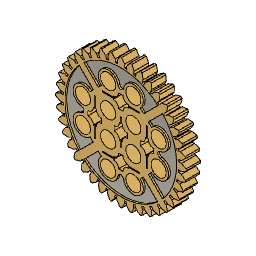
Gear_v1 (Autodesk Fusion 360 design; units mm, degrees)
Autodesk Fusion 360 part; units mm, degrees
(part 1 of 2)
sketch "Sketch1" plane through (0, 0, 0) normal (0, 1, 0) x (1, 0, 0) in component "Component"
sketch "Sketch1 (2)" plane through (0, 0, 0) normal (0, 1, 0) x (1, 0, 0)
  circle A0 centre (36.5707, -36.5204) radius 32.2395
  line L0 (34.5837, -4.281) -> (34.5837, -2.63)
  line L1 (34.5837, -2.63) -> (36.0971, -0.1323)
  line L2 (36.0971, -0.1323) -> (37.0337, -0.1323)
  line L3 (37.0337, -0.1323) -> (38.5022, -2.6935)
  line L4 (38.5022, -2.6935) -> (38.5022, -4.3286)
  line L5 (38.5022, -68.8049) -> (38.5022, -70.4559)
  line L6 (38.5022, -70.4559) -> (36.9888, -72.9536)
  line L7 (36.9888, -72.9536) -> (36.0521, -72.9536)
  line L8 (36.0521, -72.9536) -> (34.5837, -70.3924)
  line L9 (34.5837, -70.3924) -> (34.5837, -68.7599)
  line L10 (29.5619, -4.9848) -> (29.3026, -3.3549)
  line L11 (29.3026, -3.3549) -> (30.4059, -0.6509)
  line L12 (30.4059, -0.6509) -> (31.332, -0.5027)
  line L13 (31.332, -0.5027) -> (33.184, -2.8046)
  line L14 (33.184, -2.8046) -> (33.438, -4.4185)
  line L15 (43.5266, -68.1011) -> (43.7833, -69.7309)
  line L16 (43.7833, -69.7309) -> (42.6799, -72.4376)
  line L17 (42.6799, -72.4376) -> (41.7539, -72.5831)
  line L18 (41.7539, -72.5831) -> (39.9045, -70.2839)
  line L19 (39.9045, -70.2839) -> (39.6478, -68.67)
  line L20 (24.7094, -6.4638) -> (24.2014, -4.8948)
  line L21 (24.2014, -4.8948) -> (24.8682, -2.0532)
  line L22 (24.8682, -2.0532) -> (25.7598, -1.7621)
  line L23 (25.7598, -1.7621) -> (27.9479, -3.7439)
  line L24 (27.9479, -3.7439) -> (28.4506, -5.2996)
  line L25 (48.3764, -66.6221) -> (48.8871, -68.1911)
  line L26 (48.8871, -68.1911) -> (48.2177, -71.0353)
  line L27 (48.2177, -71.0353) -> (47.3287, -71.3237)
  line L28 (47.3287, -71.3237) -> (45.1406, -69.342)
  line L29 (45.1406, -69.342) -> (44.6352, -67.7889)
  line L30 (20.1507, -8.6863) -> (19.4019, -7.2152)
  line L31 (19.4019, -7.2152) -> (19.6162, -4.3021)
  line L32 (19.6162, -4.3021) -> (20.4523, -3.8788)
  line L33 (20.4523, -3.8788) -> (22.9209, -5.4928)
  line L34 (22.9209, -5.4928) -> (23.6643, -6.948)
  line L35 (52.9352, -64.3996) -> (53.684, -65.8707)
  line L36 (53.684, -65.8707) -> (53.4696, -68.7837)
  line L37 (53.4696, -68.7837) -> (52.6362, -69.2097)
  line L38 (52.6362, -69.2097) -> (50.165, -67.5931)
  line L39 (50.165, -67.5931) -> (49.4242, -66.1379)
  line L40 (15.9941, -11.594) -> (15.0257, -10.2579)
  line L41 (15.0257, -10.2579) -> (14.7823, -7.3475)
  line L42 (14.7823, -7.3475) -> (15.539, -6.7971)
  line L43 (15.539, -6.7971) -> (18.2324, -8.0063)
  line L44 (18.2324, -8.0063) -> (19.1929, -9.3292)
  line L45 (57.0918, -61.4918) -> (58.0628, -62.828)
  line L46 (58.0628, -62.828) -> (58.3062, -65.7384)
  line L47 (58.3062, -65.7384) -> (57.5469, -66.2887)
  line L48 (57.5469, -66.2887) -> (54.8561, -65.0796)
  line L49 (54.8561, -65.0796) -> (53.8956, -63.7593)
  line L50 (12.3455, -15.1156) -> (11.1786, -13.9488)
  line L51 (11.1786, -13.9488) -> (10.4828, -11.1125)
  line L52 (10.4828, -11.1125) -> (11.1442, -10.4484)
  line L53 (11.1442, -10.4484) -> (13.9938, -11.221)
  line L54 (13.9938, -11.221) -> (15.1474, -12.3772)
  line L55 (60.743, -57.9702) -> (61.9099, -59.137)
  line L56 (61.9099, -59.137) -> (62.6057, -61.976)
  line L57 (62.6057, -61.976) -> (61.9416, -62.6375)
  line L58 (61.9416, -62.6375) -> (59.0947, -61.8649)
  line L59 (59.0947, -61.8649) -> (57.9385, -60.7086)
  line L60 (9.2922, -19.1638) -> (7.956, -18.1954)
  line L61 (7.956, -18.1954) -> (6.8236, -15.5019)
  line L62 (6.8236, -15.5019) -> (7.3739, -14.7452)
  line L63 (7.3739, -14.7452) -> (10.3108, -15.0627)
  line L64 (10.3108, -15.0627) -> (11.6311, -16.0232)
  line L65 (63.7963, -53.9221) -> (65.1298, -54.8905)
  line L66 (65.1298, -54.8905) -> (66.2623, -57.5839)
  line L67 (66.2623, -57.5839) -> (65.7119, -58.3433)
  line L68 (65.7119, -58.3433) -> (62.7777, -58.0258)
  line L69 (62.7777, -58.0258) -> (61.4548, -57.0653)
  line L70 (6.9083, -23.6432) -> (5.4372, -22.8944)
  line L71 (5.4372, -22.8944) -> (3.8973, -20.41)
  line L72 (3.8973, -20.41) -> (4.3233, -19.5739)
  line L73 (4.3233, -19.5739) -> (7.2734, -19.431)
  line L74 (7.2734, -19.431) -> (8.7286, -20.1718)
  line L75 (66.1802, -49.4453) -> (67.6487, -50.1941)
  line L76 (67.6487, -50.1941) -> (69.1885, -52.6759)
  line L77 (69.1885, -52.6759) -> (68.7626, -53.512)
  line L78 (68.7626, -53.512) -> (65.8151, -53.6575)
  line L79 (65.8151, -53.6575) -> (64.3599, -52.914)
  line L80 (5.2546, -28.4374) -> (3.6856, -27.9268)
  line L81 (3.6856, -27.9268) -> (1.7754, -25.7149)
  line L82 (1.7754, -25.7149) -> (2.0664, -24.8259)
  line L83 (2.0664, -24.8259) -> (4.9556, -24.22)
  line L84 (4.9556, -24.22) -> (6.5088, -24.7253)
  line L85 (67.8339, -44.6484) -> (69.4029, -45.1591)
  line L86 (69.4029, -45.1591) -> (71.3105, -47.371)
  line L87 (71.3105, -47.371) -> (71.0195, -48.2626)
  line L88 (71.0195, -48.2626) -> (68.1302, -48.8659)
  line L89 (68.1302, -48.8659) -> (66.5771, -48.3632)
  line L90 (4.3709, -33.4328) -> (2.7411, -33.1735)
  line L91 (2.7411, -33.1735) -> (0.5106, -31.287)
  line L92 (0.5106, -31.287) -> (0.6562, -30.3609)
  line L93 (0.6562, -30.3609) -> (3.4158, -29.3132)
  line L94 (3.4158, -29.3132) -> (5.0297, -29.5672)
  line L95 (68.7149, -39.6558) -> (70.3448, -39.9124)
  line L96 (70.3448, -39.9124) -> (72.5752, -41.7989)
  line L97 (72.5752, -41.7989) -> (72.4297, -42.7249)
  line L98 (72.4297, -42.7249) -> (69.6701, -43.7727)
  line L99 (69.6701, -43.7727) -> (68.0561, -43.5187)
  line L100 (4.281, -38.5022) -> (2.63, -38.5022)
  line L101 (2.63, -38.5022) -> (0.1323, -36.9888)
  line L102 (0.1323, -36.9888) -> (0.1323, -36.0521)
  line L103 (0.1323, -36.0521) -> (2.6935, -34.5837)
  line L104 (2.6935, -34.5837) -> (4.3286, -34.5837)
  line L105 (68.8049, -34.5837) -> (70.4559, -34.5837)
  line L106 (70.4559, -34.5837) -> (72.9536, -36.0971)
  line L107 (72.9536, -36.0971) -> (72.9536, -37.0337)
  line L108 (72.9536, -37.0337) -> (70.3924, -38.5022)
  line L109 (70.3924, -38.5022) -> (68.7599, -38.5022)
  line L110 (4.9848, -43.5266) -> (3.3549, -43.7833)
  line L111 (3.3549, -43.7833) -> (0.6509, -42.6799)
  line L112 (0.6509, -42.6799) -> (0.5027, -41.7539)
  line L113 (0.5027, -41.7539) -> (2.8046, -39.9045)
  line L114 (2.8046, -39.9045) -> (4.4185, -39.6478)
  line L115 (68.1011, -29.5619) -> (69.7309, -29.3026)
  line L116 (69.7309, -29.3026) -> (72.4376, -30.4059)
  line L117 (72.4376, -30.4059) -> (72.5831, -31.332)
  line L118 (72.5831, -31.332) -> (70.2839, -33.184)
  line L119 (70.2839, -33.184) -> (68.67, -33.438)
  line L120 (6.4638, -48.3764) -> (4.8948, -48.8871)
  line L121 (4.8948, -48.8871) -> (2.0532, -48.2177)
  line L122 (2.0532, -48.2177) -> (1.7621, -47.3287)
  line L123 (1.7621, -47.3287) -> (3.7439, -45.1406)
  line L124 (3.7439, -45.1406) -> (5.2996, -44.6352)
  line L125 (66.6221, -24.7094) -> (68.1911, -24.2014)
  line L126 (68.1911, -24.2014) -> (71.0353, -24.8682)
  line L127 (71.0353, -24.8682) -> (71.3237, -25.7598)
  line L128 (71.3237, -25.7598) -> (69.342, -27.9479)
  line L129 (69.342, -27.9479) -> (67.7889, -28.4506)
  line L130 (8.6863, -52.9352) -> (7.2152, -53.684)
  line L131 (7.2152, -53.684) -> (4.3021, -53.4696)
  line L132 (4.3021, -53.4696) -> (3.8788, -52.6362)
  line L133 (3.8788, -52.6362) -> (5.4928, -50.165)
  line L134 (5.4928, -50.165) -> (6.948, -49.4242)
  line L135 (64.3996, -20.1507) -> (65.8707, -19.4019)
  line L136 (65.8707, -19.4019) -> (68.7837, -19.6162)
  line L137 (68.7837, -19.6162) -> (69.2097, -20.4523)
  line L138 (69.2097, -20.4523) -> (67.5931, -22.9209)
  line L139 (67.5931, -22.9209) -> (66.1379, -23.6643)
  line L140 (11.594, -57.0918) -> (10.2579, -58.0628)
  line L141 (10.2579, -58.0628) -> (7.3475, -58.3062)
  line L142 (7.3475, -58.3062) -> (6.7971, -57.5469)
  line L143 (6.7971, -57.5469) -> (8.0063, -54.8561)
  line L144 (8.0063, -54.8561) -> (9.3292, -53.8956)
  line L145 (61.4918, -15.9941) -> (62.828, -15.0257)
  line L146 (62.828, -15.0257) -> (65.7384, -14.7823)
  line L147 (65.7384, -14.7823) -> (66.2887, -15.539)
  line L148 (66.2887, -15.539) -> (65.0796, -18.2324)
  line L149 (65.0796, -18.2324) -> (63.7593, -19.1929)
  line L150 (15.1156, -60.743) -> (13.9488, -61.9099)
  line L151 (13.9488, -61.9099) -> (11.1125, -62.6057)
  line L152 (11.1125, -62.6057) -> (10.4484, -61.9416)
  line L153 (10.4484, -61.9416) -> (11.221, -59.0947)
  line L154 (11.221, -59.0947) -> (12.3772, -57.9385)
  line L155 (57.9702, -12.3455) -> (59.137, -11.1786)
  line L156 (59.137, -11.1786) -> (61.976, -10.4828)
  line L157 (61.976, -10.4828) -> (62.6375, -11.1442)
  line L158 (62.6375, -11.1442) -> (61.8649, -13.9938)
  line L159 (61.8649, -13.9938) -> (60.7086, -15.1474)
  line L160 (19.1638, -63.7963) -> (18.1954, -65.1298)
  line L161 (18.1954, -65.1298) -> (15.5019, -66.2623)
  line L162 (15.5019, -66.2623) -> (14.7452, -65.7119)
  line L163 (14.7452, -65.7119) -> (15.0627, -62.7777)
  line L164 (15.0627, -62.7777) -> (16.0232, -61.4548)
  line L165 (53.9221, -9.2922) -> (54.8905, -7.956)
  line L166 (54.8905, -7.956) -> (57.5839, -6.8236)
  line L167 (57.5839, -6.8236) -> (58.3433, -7.3739)
  line L168 (58.3433, -7.3739) -> (58.0258, -10.3108)
  line L169 (58.0258, -10.3108) -> (57.0653, -11.6311)
  line L170 (23.6432, -66.1802) -> (22.8944, -67.6487)
  line L171 (22.8944, -67.6487) -> (20.41, -69.1885)
  line L172 (20.41, -69.1885) -> (19.5739, -68.7626)
  line L173 (19.5739, -68.7626) -> (19.431, -65.8151)
  line L174 (19.431, -65.8151) -> (20.1718, -64.3599)
  line L175 (49.4453, -6.9083) -> (50.1941, -5.4372)
  line L176 (50.1941, -5.4372) -> (52.6759, -3.8973)
  line L177 (52.6759, -3.8973) -> (53.512, -4.3233)
  line L178 (53.512, -4.3233) -> (53.6575, -7.2734)
  line L179 (53.6575, -7.2734) -> (52.914, -8.7286)
  line L180 (28.4374, -67.8339) -> (27.9268, -69.4029)
  line L181 (27.9268, -69.4029) -> (25.7149, -71.3105)
  line L182 (25.7149, -71.3105) -> (24.8259, -71.0195)
  line L183 (24.8259, -71.0195) -> (24.22, -68.1302)
  line L184 (24.22, -68.1302) -> (24.7253, -66.5771)
  line L185 (44.6484, -5.2546) -> (45.1591, -3.6856)
  line L186 (45.1591, -3.6856) -> (47.371, -1.7754)
  line L187 (47.371, -1.7754) -> (48.2626, -2.0664)
  line L188 (48.2626, -2.0664) -> (48.8659, -4.9556)
  line L189 (48.8659, -4.9556) -> (48.3632, -6.5088)
  line L190 (33.4328, -68.7149) -> (33.1735, -70.3448)
  line L191 (33.1735, -70.3448) -> (31.287, -72.5752)
  line L192 (31.287, -72.5752) -> (30.3609, -72.4297)
  line L193 (30.3609, -72.4297) -> (29.3132, -69.6701)
  line L194 (29.3132, -69.6701) -> (29.5672, -68.0561)
  line L195 (39.6558, -4.3709) -> (39.9124, -2.7411)
  line L196 (39.9124, -2.7411) -> (41.7989, -0.5106)
  line L197 (41.7989, -0.5106) -> (42.7249, -0.6562)
  line L198 (42.7249, -0.6562) -> (43.7727, -3.4158)
  line L199 (43.7727, -3.4158) -> (43.5187, -5.0297)
  circle A1 centre (43.7727, -29.3132) radius 4.019
  circle A2 centre (43.7727, -15.9015) radius 4.019
  circle A3 centre (43.7727, -57.1315) radius 4.019
  circle A4 centre (43.7727, -43.6219) radius 4.019
  circle A5 centre (57.1844, -29.3132) radius 4.019
  circle A6 centre (57.1844, -43.6219) radius 4.019
  circle A7 centre (29.8371, -29.3158) radius 4.019
  circle A8 centre (29.8371, -15.9041) radius 4.019
  circle A9 centre (29.8371, -57.1341) radius 4.019
  circle A10 centre (29.8371, -43.6245) radius 4.019
  circle A11 centre (16.4253, -29.3158) radius 4.019
  circle A12 centre (16.4253, -43.6245) radius 4.019
  line L200 (47.0667, -22.6166) -> (40.6162, -22.6166)
  line L201 (40.6162, -22.6166) -> (40.6162, -21.9181)
  arc A13 (40.6162, -21.9181) -> (37.9889, -19.2908) centre (40.6188, -19.2881) cw
  spline S0 degree 3 poles (37.9889, -19.2908) (37.9889, -19.2458) (37.9889, -19.2035) (37.9889, -19.1585) knots 0 0 0 0 1 1 1 1
  line L202 (37.9889, -19.1585) -> (35.5283, -19.1585)
  arc A14 (35.5283, -19.1585) -> (32.9009, -21.7858) centre (32.8983, -19.1558) cw
  line L203 (32.9009, -21.7858) -> (32.9009, -22.6166)
  line L204 (32.9009, -22.6166) -> (26.4504, -22.6166)
  arc A15 (26.3181, -22.7489) -> (26.4504, -22.6166) centre (26.4504, -22.7489) cw
  line L205 (26.3181, -22.7489) -> (26.3181, -23.278)
  arc A16 (26.4504, -23.4103) -> (26.3181, -23.278) centre (26.4504, -23.278) cw
  line L206 (26.4504, -23.4103) -> (32.9009, -23.4103)
  line L207 (32.9009, -23.4103) -> (32.9009, -24.2438)
  arc A17 (32.9009, -24.2438) -> (35.5283, -26.8711) centre (32.8983, -26.8737) cw
  line L208 (35.5283, -26.8711) -> (37.9809, -26.8711)
  arc A18 (37.9809, -26.8711) -> (40.6083, -24.2438) centre (40.6109, -26.8737) cw
  line L209 (40.6083, -24.2438) -> (40.6083, -23.413)
  line L210 (40.6083, -23.413) -> (47.0588, -23.413)
  arc A19 (47.1911, -23.2807) -> (47.0588, -23.413) centre (47.0588, -23.2807) cw
  line L211 (47.1911, -23.2807) -> (47.1911, -22.7515)
  arc A20 (47.0667, -22.6166) -> (47.1911, -22.7515) centre (47.0588, -22.7486) cw
  line L212 (47.0667, -50.3026) -> (40.6162, -50.3026)
  line L213 (40.6162, -50.3026) -> (40.6162, -49.6014)
  arc A21 (40.6162, -49.6014) -> (37.9889, -46.9741) centre (40.6162, -46.9741) cw
  spline S1 degree 3 poles (37.9889, -46.9741) (37.9889, -46.9291) (37.9889, -46.8868) (37.9889, -46.8418) knots 0 0 0 0 1 1 1 1
  line L214 (37.9889, -46.8418) -> (35.5283, -46.8418)
  arc A22 (35.5283, -46.8418) -> (32.9009, -49.4691) centre (32.9009, -46.8418) cw
  line L215 (32.9009, -49.4691) -> (32.9009, -50.3026)
  line L216 (32.9009, -50.3026) -> (26.4504, -50.3026)
  arc A23 (26.3181, -50.4349) -> (26.4504, -50.3026) centre (26.4504, -50.4349) cw
  line L217 (26.3181, -50.4349) -> (26.3181, -50.964)
  arc A24 (26.4504, -51.0963) -> (26.3181, -50.964) centre (26.4504, -50.964) cw
  line L218 (26.4504, -51.0963) -> (32.9009, -51.0963)
  line L219 (32.9009, -51.0963) -> (32.9009, -51.9298)
  arc A25 (32.9009, -51.9298) -> (35.5283, -54.5571) centre (32.9009, -54.5571) cw
  line L220 (35.5283, -54.5571) -> (37.9809, -54.5571)
  arc A26 (37.9809, -54.5571) -> (40.6083, -51.9298) centre (40.6083, -54.5571) cw
  line L221 (40.6083, -51.9298) -> (40.6083, -51.0963)
  line L222 (40.6083, -51.0963) -> (47.0588, -51.0963)
  arc A27 (47.1911, -50.964) -> (47.0588, -51.0963) centre (47.0588, -50.964) cw
  line L223 (47.1911, -50.964) -> (47.1911, -50.4349)
  arc A28 (47.0667, -50.3026) -> (47.1911, -50.4349) centre (47.0588, -50.4346) cw
  line L224 (22.5266, -26.5509) -> (22.5266, -33.0015)
  line L225 (22.5266, -33.0015) -> (21.8255, -33.0015)
  arc A29 (21.8255, -33.0015) -> (19.1982, -35.6261) centre (19.1982, -32.9988) cw
  line L226 (19.1982, -35.6261) -> (19.0659, -35.6261)
  line L227 (19.0659, -35.6261) -> (19.0659, -38.0868)
  arc A30 (19.0659, -38.0868) -> (21.6932, -40.7141) centre (19.0632, -40.7167) cw
  line L228 (21.6932, -40.7141) -> (22.5266, -40.7141)
  line L229 (22.5266, -40.7141) -> (22.5266, -47.1646)
  arc A31 (22.6589, -47.2969) -> (22.5266, -47.1646) centre (22.6589, -47.1646) cw
  line L230 (22.6589, -47.2969) -> (23.1881, -47.2969)
  arc A32 (23.3204, -47.1646) -> (23.1881, -47.2969) centre (23.1881, -47.1646) cw
  line L231 (23.3204, -47.1646) -> (23.3204, -40.7088)
  line L232 (23.3204, -40.7088) -> (24.1538, -40.7088)
  arc A33 (24.1538, -40.7088) -> (26.7811, -38.0815) centre (26.7811, -40.7088) cw
  line L233 (26.7811, -38.0815) -> (26.7811, -35.6209)
  arc A34 (26.7811, -35.6209) -> (24.1538, -32.9962) centre (26.7785, -32.9962) cw
  line L234 (24.1538, -32.9962) -> (23.3204, -32.9962)
  line L235 (23.3204, -32.9962) -> (23.3204, -26.5509)
  arc A35 (23.1881, -26.4186) -> (23.3204, -26.5509) centre (23.1881, -26.5509) cw
  line L236 (23.1881, -26.4186) -> (22.6589, -26.4186)
  arc A36 (22.5266, -26.5509) -> (22.6589, -26.4186) centre (22.6589, -26.5509) cw
  line L237 (50.21, -26.5509) -> (50.21, -33.0015)
  line L238 (50.21, -33.0015) -> (49.5088, -33.0015)
  arc A37 (49.5088, -33.0015) -> (46.8815, -35.6261) centre (46.8842, -33.0015) cw
  line L239 (46.8815, -35.6261) -> (46.7492, -35.6261)
  line L240 (46.7492, -35.6261) -> (46.7492, -38.0868)
  arc A38 (46.7492, -38.0868) -> (49.3765, -40.7141) centre (46.7492, -40.7141) cw
  line L241 (49.3765, -40.7141) -> (50.21, -40.7141)
  line L242 (50.21, -40.7141) -> (50.21, -47.1646)
  arc A39 (50.3423, -47.2969) -> (50.21, -47.1646) centre (50.3423, -47.1646) cw
  line L243 (50.3423, -47.2969) -> (50.8714, -47.2969)
  arc A40 (51.0037, -47.1646) -> (50.8714, -47.2969) centre (50.8714, -47.1646) cw
  line L244 (51.0037, -47.1646) -> (51.0037, -40.7088)
  line L245 (51.0037, -40.7088) -> (51.8372, -40.7088)
  arc A41 (51.8372, -40.7088) -> (54.4645, -38.0815) centre (54.4645, -40.7088) cw
  line L246 (54.4645, -38.0815) -> (54.4645, -35.6209)
  arc A42 (54.4645, -35.6209) -> (51.8372, -32.9962) centre (54.4618, -32.9962) cw
  line L247 (51.8372, -32.9962) -> (51.0037, -32.9962)
  line L248 (51.0037, -32.9962) -> (51.0037, -26.5509)
  arc A43 (50.8714, -26.4186) -> (51.0037, -26.5509) centre (50.8714, -26.5509) cw
  line L249 (50.8714, -26.4186) -> (50.3423, -26.4186)
  arc A44 (50.21, -26.5509) -> (50.3423, -26.4186) centre (50.3423, -26.5509) cw
  line L250 (37.7984, -32.6893) -> (37.3327, -32.6893)
  line L251 (37.3327, -32.6893) -> (37.3327, -28.5591)
  arc A45 (37.2004, -28.4268) -> (37.3327, -28.5591) centre (37.1978, -28.5617) cw
  line L252 (37.2004, -28.4268) -> (36.105, -28.4268)
  arc A46 (35.9727, -28.5591) -> (36.105, -28.4268) centre (36.1077, -28.5617) cw
  line L253 (35.9727, -28.5591) -> (35.9727, -32.6893)
  line L254 (35.9727, -32.6893) -> (35.478, -32.6893)
  arc A47 (35.478, -32.6893) -> (32.8507, -35.3166) centre (32.848, -32.6866) cw
  spline S2 degree 3 poles (32.8507, -35.3166) (32.8057, -35.3166) (32.7607, -35.3166) (32.7184, -35.3166) knots 0 0 0 0 1 1 1 1
  line L255 (32.7184, -35.3166) -> (32.7184, -37.7799)
  arc A48 (32.7184, -37.7799) -> (35.3457, -40.4045) centre (32.7184, -40.4072) cw
  line L256 (35.3457, -40.4045) -> (35.9727, -40.4045)
  line L257 (35.9727, -40.4045) -> (35.9727, -44.487)
  arc A49 (36.105, -44.6193) -> (35.9727, -44.487) centre (36.105, -44.487) cw
  line L258 (36.105, -44.6193) -> (37.2136, -44.6193)
  arc A50 (37.3459, -44.487) -> (37.2136, -44.6193) centre (37.2136, -44.487) cw
  line L259 (37.3459, -44.487) -> (37.3459, -40.3966)
  line L260 (37.3459, -40.3966) -> (37.8116, -40.3966)
  arc A51 (37.8116, -40.3966) -> (40.4389, -37.7719) centre (40.4389, -40.3992) cw
  line L261 (40.4389, -37.7719) -> (40.4389, -35.3166)
  arc A52 (40.4389, -35.3166) -> (37.7984, -32.6893) centre (40.4283, -32.6866) cw
  circle A53 centre (29.6466, -15.9041) radius 4.019
  arc A54 (48.9982, -15.8935) -> (47.4689, -19.5977) centre (43.778, -15.9061) cw
  arc A55 (43.7727, -10.668) -> (48.9982, -15.8935) centre (43.7727, -15.8935) cw
  arc A56 (38.5366, -15.9015) -> (43.7727, -10.668) centre (43.7621, -15.8935) cw
  spline S3 degree 3 poles (38.5366, -15.9015) (38.5366, -16.0734) (38.5366, -16.2428) (38.563, -16.4095) knots 0 0 0 0 1 1 1 1
  arc A57 (43.7621, -62.357) -> (38.5366, -57.1315) centre (43.7621, -57.1315) cw
  arc A58 (48.9876, -57.1315) -> (43.7621, -62.357) centre (43.7621, -57.1315) cw
  arc A59 (47.4451, -53.4273) -> (48.9876, -57.1315) centre (43.7833, -57.1255) cw
  arc A60 (62.4099, -29.3132) -> (57.1844, -34.5387) centre (57.1844, -29.3132) cw
  arc A61 (57.1844, -24.0877) -> (62.4099, -29.3132) centre (57.1844, -29.3132) cw
  arc A62 (53.4802, -25.617) -> (57.1844, -24.0877) centre (57.1674, -29.2973) cw
  arc A63 (57.1844, -48.85) -> (53.504, -47.3287) centre (57.1811, -43.6457) cw
  arc A64 (62.4099, -43.6245) -> (57.1844, -48.85) centre (57.1844, -43.6245) cw
  arc A65 (57.1844, -38.399) -> (62.4099, -43.6245) centre (57.1844, -43.6245) cw
  arc A66 (24.421, -57.1341) -> (25.7784, -53.631) centre (29.6175, -57.133) cw
  arc A67 (29.6466, -62.3596) -> (24.421, -57.1341) centre (29.6466, -57.1341) cw
  arc A68 (34.8721, -57.1659) -> (29.6466, -62.3596) centre (29.6467, -57.1341) cw
  arc A69 (16.4174, -24.0903) -> (20.1216, -25.6222) centre (16.4328, -29.2973) cw
  arc A70 (11.1919, -29.3158) -> (16.4174, -24.0903) centre (16.4174, -29.3158) cw
  arc A71 (16.4174, -34.5414) -> (11.1919, -29.3158) centre (16.4174, -29.3158) cw
  arc A72 (11.1998, -43.6245) -> (16.4253, -38.399) centre (16.4253, -43.6245) cw
  arc A73 (16.4253, -48.85) -> (11.1998, -43.6245) centre (16.4253, -43.6245) cw
  arc A74 (20.029, -47.4027) -> (16.4253, -48.85) centre (16.4287, -43.6483) cw
  arc A75 (29.6466, -10.6786) -> (34.8721, -15.9041) centre (29.6466, -15.9041) cw
  arc A76 (24.421, -15.9041) -> (29.6466, -10.6786) centre (29.6466, -15.9041) cw
  arc A77 (26.0509, -19.6903) -> (24.421, -15.9041) centre (29.6254, -15.9077) cw
  line L262 (26.0509, -19.6903) -> (20.1216, -25.6222)
  line L263 (47.4689, -19.5977) -> (53.4908, -25.617)
  line L264 (47.4557, -53.422) -> (53.504, -47.3287)
  line L265 (25.9689, -53.631) -> (20.029, -47.4027)
  spline S4 degree 3 poles (34.9065, -15.9041) (34.9065, -17.0154) (35.6579, -17.9123) (36.5892, -17.9202) knots 0 0 0 0 1 1 1 1
  line L266 (36.5892, -17.9202) -> (36.6025, -17.9202)
  spline S5 degree 3 poles (36.5892, -17.9202) (37.6211, -17.9202) (38.4651, -17.2561) (38.5736, -16.4095) knots 0 0 0 0 1 1 1 1
  line L267 (36.5892, -17.9202) -> (36.5707, -17.9202)
  arc A78 (38.5868, -16.2243) -> (38.5736, -16.4095) centre (37.1687, -16.2161) cw
  spline S6 degree 3 poles (38.5868, -58.1395) (38.5868, -57.0309) (37.8354, -56.134) (36.9014, -56.1234) knots 0 0 0 0 1 1 1 1
  line L268 (36.8882, -56.1234) -> (36.9014, -56.1234)
  arc A79 (34.9065, -57.8194) -> (35.0626, -57.1659) centre (36.3643, -57.8222) cw
  arc A80 (35.0494, -57.1659) -> (36.9014, -56.1234) centre (36.8325, -58.1675) cw
  line L269 (36.9014, -56.1234) -> (36.9226, -56.1234)
  spline S7 degree 3 poles (15.6289, -38.2905) (16.7375, -38.2905) (17.6345, -37.5391) (17.6451, -36.6077) knots 0 0 0 0 1 1 1 1
  line L270 (17.6345, -36.6263) -> (17.6345, -36.6077)
  spline S8 degree 3 poles (15.9464, -34.6101) (16.8804, -34.6101) (17.6345, -35.5018) (17.6451, -36.6077) knots 0 0 0 0 1 1 1 1
  spline S9 degree 3 poles (57.6712, -34.6101) (56.5626, -34.6101) (55.6657, -35.3616) (55.6578, -36.2955) knots 0 0 0 0 1 1 1 1
  spline S10 degree 2 poles (55.8456, -36.2744) (55.8456, -36.2876) (55.8456, -36.2955) knots 0 0 0 1 1 1
  spline S11 degree 3 poles (57.3537, -38.2905) (56.4197, -38.2905) (55.6657, -37.3989) (55.6578, -36.2955) knots 0 0 0 0 1 1 1 1
  arc A81 (59.5551, -16.2481) -> (67.228, -36.5204) centre (36.7215, -36.4786) cw
  arc A82 (67.228, -36.5204) -> (59.4942, -56.8616) centre (36.7215, -36.5626) cw
  line L271 (59.4942, -56.8616) -> (51.7393, -49.1146)
  arc A83 (36.6025, -5.8949) -> (56.8563, -13.552) centre (36.6457, -36.3961) cw
  arc A84 (16.2613, -13.6287) -> (36.6025, -5.8949) centre (36.5603, -36.4013) cw
  line L272 (16.2613, -13.6287) -> (24.1988, -21.5662)
  line L273 (56.8563, -13.552) -> (49.1384, -21.2672)
  line L274 (59.5551, -16.2481) -> (51.8372, -23.966)
  line L275 (21.4895, -24.2438) -> (13.5731, -16.3274)
  arc A85 (5.9928, -36.5204) -> (13.5731, -16.3274) centre (36.486, -36.4481) cw
  arc A86 (13.6472, -56.7716) -> (5.9928, -36.5204) centre (36.4966, -36.563) cw
  line L276 (13.6472, -56.7716) -> (21.4947, -48.9241)
  line L277 (24.1141, -51.689) -> (16.3301, -59.473)
  arc A87 (36.6025, -67.146) -> (16.3301, -59.473) centre (36.5636, -36.6316) cw
  arc A88 (56.7928, -59.5498) -> (36.6025, -67.146) centre (36.6542, -36.6528) cw
  line L278 (56.7928, -59.5498) -> (49.059, -51.816)
  line L279 (20.1216, -25.6222) -> (21.4895, -24.2544)
  line L280 (21.4895, -24.2544) -> (26.0509, -19.6903)
  circle A89 centre (313.1582, -43.7383) radius 32.2395
  line L281 (311.1738, -11.4988) -> (311.1738, -9.8478)
  line L282 (311.1738, -9.8478) -> (312.6872, -7.3501)
  line L283 (312.6872, -7.3501) -> (313.6239, -7.3501)
  line L284 (313.6239, -7.3501) -> (315.0923, -9.9113)
  line L285 (315.0923, -9.9113) -> (315.0923, -11.5438)
  line L286 (315.0923, -76.0227) -> (315.0923, -77.6737)
  line L287 (315.0923, -77.6737) -> (313.5762, -80.1714)
  line L288 (313.5762, -80.1714) -> (312.6396, -80.1714)
  line L289 (312.6396, -80.1714) -> (311.1738, -77.6102)
  line L290 (311.1738, -77.6102) -> (311.1738, -75.9751)
  line L291 (306.1494, -12.2026) -> (305.8927, -10.5728)
  line L292 (305.8927, -10.5728) -> (306.996, -7.8661)
  line L293 (306.996, -7.8661) -> (307.9221, -7.7205)
  line L294 (307.9221, -7.7205) -> (309.7715, -10.0198)
  line L295 (309.7715, -10.0198) -> (310.0282, -11.6337)
  line L296 (320.1141, -75.3189) -> (320.3734, -76.9488)
  line L297 (320.3734, -76.9488) -> (319.2674, -79.6528)
  line L298 (319.2674, -79.6528) -> (318.3414, -79.801)
  line L299 (318.3414, -79.801) -> (316.4919, -77.4991)
  line L300 (316.4919, -77.4991) -> (316.2353, -75.8851)
  line L301 (301.2996, -13.6816) -> (300.7889, -12.1126)
  line L302 (300.7889, -12.1126) -> (301.4557, -9.2684)
  line L303 (301.4557, -9.2684) -> (302.3473, -8.98)
  line L304 (302.3473, -8.98) -> (304.5354, -10.9617)
  line L305 (304.5354, -10.9617) -> (305.0408, -12.5148)
  line L306 (324.9639, -73.8373) -> (325.4745, -75.4063)
  line L307 (325.4745, -75.4063) -> (324.8078, -78.2505)
  line L308 (324.8078, -78.2505) -> (323.9161, -78.5416)
  line L309 (323.9161, -78.5416) -> (321.728, -76.5598)
  line L310 (321.728, -76.5598) -> (321.2253, -75.0041)
  line L311 (296.7381, -15.9041) -> (295.9894, -14.433)
  line L312 (295.9894, -14.433) -> (296.2037, -11.52)
  line L313 (296.2037, -11.52) -> (297.0398, -11.094)
  line L314 (297.0398, -11.094) -> (299.511, -12.7106)
  line L315 (299.511, -12.7106) -> (300.2518, -14.1658)
  line L316 (329.5253, -71.6174) -> (330.2741, -73.0885)
  line L317 (330.2741, -73.0885) -> (330.0598, -76.0016)
  line L318 (330.0598, -76.0016) -> (329.2237, -76.4249)
  line L319 (329.2237, -76.4249) -> (326.7525, -74.8109)
  line L320 (326.7525, -74.8109) -> (326.0116, -73.3557)
  line L321 (292.5842, -18.8119) -> (291.6132, -17.4757)
  line L322 (291.6132, -17.4757) -> (291.3698, -14.5653)
  line L323 (291.3698, -14.5653) -> (292.1265, -14.015)
  line L324 (292.1265, -14.015) -> (294.8199, -15.2241)
  line L325 (294.8199, -15.2241) -> (295.7804, -16.5444)
  line L326 (333.6793, -68.7096) -> (334.6503, -70.0458)
  line L327 (334.6503, -70.0458) -> (334.8937, -72.9562)
  line L328 (334.8937, -72.9562) -> (334.137, -73.5065)
  line L329 (334.137, -73.5065) -> (331.4435, -72.2974)
  line L330 (331.4435, -72.2974) -> (330.4831, -70.9745)
  line L331 (288.9329, -22.3335) -> (287.7661, -21.1667)
  line L332 (287.7661, -21.1667) -> (287.0703, -18.3303)
  line L333 (287.0703, -18.3303) -> (287.7317, -17.6662)
  line L334 (287.7317, -17.6662) -> (290.5813, -18.4388)
  line L335 (290.5813, -18.4388) -> (291.7375, -19.595)
  line L336 (337.3305, -65.188) -> (338.4973, -66.3549)
  line L337 (338.4973, -66.3549) -> (339.1932, -69.1912)
  line L338 (339.1932, -69.1912) -> (338.5317, -69.8553)
  line L339 (338.5317, -69.8553) -> (335.6822, -69.0827)
  line L340 (335.6822, -69.0827) -> (334.5259, -67.9265)
  line L341 (285.8796, -26.3816) -> (284.5435, -25.4132)
  line L342 (284.5435, -25.4132) -> (283.4137, -22.7198)
  line L343 (283.4137, -22.7198) -> (283.9641, -21.9604)
  line L344 (283.9641, -21.9604) -> (286.8983, -22.2779)
  line L345 (286.8983, -22.2779) -> (288.2212, -23.2384)
  line L346 (340.3838, -61.1399) -> (341.72, -62.1083)
  line L347 (341.72, -62.1083) -> (342.8524, -64.8017)
  line L348 (342.8524, -64.8017) -> (342.2994, -65.5585)
  line L349 (342.2994, -65.5585) -> (339.3652, -65.241)
  line L350 (339.3652, -65.241) -> (338.0449, -64.2805)
  line L351 (283.4958, -30.8584) -> (282.0273, -30.1096)
  line L352 (282.0273, -30.1096) -> (280.4874, -27.6278)
  line L353 (280.4874, -27.6278) -> (280.9134, -26.7917)
  line L354 (280.9134, -26.7917) -> (283.8609, -26.6462)
  line L355 (283.8609, -26.6462) -> (285.3161, -27.3897)
  line L356 (342.7677, -56.6605) -> (344.2388, -57.4119)
  line L357 (344.2388, -57.4119) -> (345.776, -59.8937)
  line L358 (345.776, -59.8937) -> (345.3527, -60.7298)
  line L359 (345.3527, -60.7298) -> (342.4026, -60.8727)
  line L360 (342.4026, -60.8727) -> (340.9474, -60.1319)
  line L361 (281.8421, -35.6526) -> (280.2731, -35.1446)
  line L362 (280.2731, -35.1446) -> (278.3655, -32.9327)
  line L363 (278.3655, -32.9327) -> (278.6539, -32.041)
  line L364 (278.6539, -32.041) -> (281.5431, -31.4378)
  line L365 (281.5431, -31.4378) -> (283.0989, -31.9405)
  line L366 (344.4214, -51.8663) -> (345.9903, -52.3769)
  line L367 (345.9903, -52.3769) -> (347.898, -54.5888)
  line L368 (347.898, -54.5888) -> (347.6096, -55.4805)
  line L369 (347.6096, -55.4805) -> (344.7203, -56.0837)
  line L370 (344.7203, -56.0837) -> (343.1672, -55.5784)
  line L371 (280.961, -40.6479) -> (279.3312, -40.3913)
  line L372 (279.3312, -40.3913) -> (277.1008, -38.5048)
  line L373 (277.1008, -38.5048) -> (277.2463, -37.5788)
  line L374 (277.2463, -37.5788) -> (280.0059, -36.531)
  line L375 (280.0059, -36.531) -> (281.6199, -36.785)
  line L376 (345.3051, -46.8736) -> (346.9323, -47.1302)
  line L377 (346.9323, -47.1302) -> (349.1653, -49.0167)
  line L378 (349.1653, -49.0167) -> (349.0172, -49.9428)
  line L379 (349.0172, -49.9428) -> (346.2576, -50.9905)
  line L380 (346.2576, -50.9905) -> (344.6463, -50.7339)
  line L381 (280.8684, -45.72) -> (279.2201, -45.72)
  line L382 (279.2201, -45.72) -> (276.7198, -44.2066)
  line L383 (276.7198, -44.2066) -> (276.7198, -43.27)
  line L384 (276.7198, -43.27) -> (279.2809, -41.8015)
  line L385 (279.2809, -41.8015) -> (280.9161, -41.8015)
  line L386 (345.395, -41.8015) -> (347.0434, -41.8015)
  line L387 (347.0434, -41.8015) -> (349.5437, -43.3149)
  line L388 (349.5437, -43.3149) -> (349.5437, -44.2516)
  line L389 (349.5437, -44.2516) -> (346.9825, -45.72)
  line L390 (346.9825, -45.72) -> (345.3474, -45.72)
  line L391 (281.5722, -50.7418) -> (279.9424, -51.0011)
  line L392 (279.9424, -51.0011) -> (277.2384, -49.8978)
  line L393 (277.2384, -49.8978) -> (277.0928, -48.9717)
  line L394 (277.0928, -48.9717) -> (279.3921, -47.1196)
  line L395 (279.3921, -47.1196) -> (281.006, -46.8656)
  line L396 (344.6912, -36.7771) -> (346.3211, -36.5204)
  line L397 (346.3211, -36.5204) -> (349.0251, -37.6238)
  line L398 (349.0251, -37.6238) -> (349.1706, -38.5498)
  line L399 (349.1706, -38.5498) -> (346.8714, -40.3992)
  line L400 (346.8714, -40.3992) -> (345.2574, -40.6559)
  line L401 (283.0539, -55.5943) -> (281.4849, -56.1023)
  line L402 (281.4849, -56.1023) -> (278.6406, -55.4355)
  line L403 (278.6406, -55.4355) -> (278.3523, -54.5439)
  line L404 (278.3523, -54.5439) -> (280.334, -52.3584)
  line L405 (280.334, -52.3584) -> (281.8871, -51.853)
  line L406 (343.2096, -31.9273) -> (344.7785, -31.4166)
  line L407 (344.7785, -31.4166) -> (347.6228, -32.086)
  line L408 (347.6228, -32.086) -> (347.9139, -32.975)
  line L409 (347.9139, -32.975) -> (345.9295, -35.1631)
  line L410 (345.9295, -35.1631) -> (344.3764, -35.6685)
  line L411 (285.2738, -60.153) -> (283.8053, -60.9018)
  line L412 (283.8053, -60.9018) -> (280.8923, -60.6875)
  line L413 (280.8923, -60.6875) -> (280.4663, -59.854)
  line L414 (280.4663, -59.854) -> (282.0829, -57.3828)
  line L415 (282.0829, -57.3828) -> (283.5381, -56.6394)
  line L416 (340.9897, -27.3685) -> (342.4581, -26.6197)
  line L417 (342.4581, -26.6197) -> (345.3712, -26.834)
  line L418 (345.3712, -26.834) -> (345.7972, -27.6675)
  line L419 (345.7972, -27.6675) -> (344.1832, -30.1387)
  line L420 (344.1832, -30.1387) -> (342.7254, -30.8795)
  line L421 (288.1815, -64.3096) -> (286.848, -65.278)
  line L422 (286.848, -65.278) -> (283.9376, -65.5241)
  line L423 (283.9376, -65.5241) -> (283.3873, -64.7647)
  line L424 (283.3873, -64.7647) -> (284.5938, -62.0713)
  line L425 (284.5938, -62.0713) -> (285.9167, -61.1108)
  line L426 (338.0819, -23.2119) -> (339.4154, -22.2409)
  line L427 (339.4154, -22.2409) -> (342.3285, -21.9975)
  line L428 (342.3285, -21.9975) -> (342.8788, -22.7568)
  line L429 (342.8788, -22.7568) -> (341.6697, -25.4503)
  line L430 (341.6697, -25.4503) -> (340.3468, -26.4081)
  line L431 (291.7031, -67.9582) -> (290.539, -69.125)
  line L432 (290.539, -69.125) -> (287.7, -69.8209)
  line L433 (287.7, -69.8209) -> (287.0385, -69.1594)
  line L434 (287.0385, -69.1594) -> (287.8111, -66.3099)
  line L435 (287.8111, -66.3099) -> (288.9673, -65.1563)
  line L436 (334.5603, -19.5606) -> (335.7271, -18.3965)
  line L437 (335.7271, -18.3965) -> (338.5635, -17.698)
  line L438 (338.5635, -17.698) -> (339.2249, -18.3621)
  line L439 (339.2249, -18.3621) -> (338.4524, -21.209)
  line L440 (338.4524, -21.209) -> (337.2988, -22.3652)
  line L441 (295.7539, -71.0142) -> (294.7829, -72.3477)
  line L442 (294.7829, -72.3477) -> (292.0894, -73.4801)
  line L443 (292.0894, -73.4801) -> (291.3327, -72.9298)
  line L444 (291.3327, -72.9298) -> (291.6502, -69.9929)
  line L445 (291.6502, -69.9929) -> (292.6106, -68.6726)
  line L446 (330.5096, -16.5074) -> (331.4806, -15.1739)
  line L447 (331.4806, -15.1739) -> (334.174, -14.0414)
  line L448 (334.174, -14.0414) -> (334.9308, -14.5918)
  line L449 (334.9308, -14.5918) -> (334.6132, -17.526)
  line L450 (334.6132, -17.526) -> (333.6528, -18.8489)
  line L451 (300.2306, -73.3954) -> (299.4819, -74.8665)
  line L452 (299.4819, -74.8665) -> (297.0001, -76.4037)
  line L453 (297.0001, -76.4037) -> (296.164, -75.9804)
  line L454 (296.164, -75.9804) -> (296.0185, -73.0303)
  line L455 (296.0185, -73.0303) -> (296.7593, -71.5751)
  line L456 (326.0328, -14.1235) -> (326.7816, -12.655)
  line L457 (326.7816, -12.655) -> (329.266, -11.1151)
  line L458 (329.266, -11.1151) -> (330.0995, -11.5411)
  line L459 (330.0995, -11.5411) -> (330.245, -14.4886)
  line L460 (330.245, -14.4886) -> (329.5041, -15.9464)
  line L461 (305.0249, -75.0491) -> (304.5169, -76.618)
  line L462 (304.5169, -76.618) -> (302.305, -78.5283)
  line L463 (302.305, -78.5283) -> (301.4133, -78.2373)
  line L464 (301.4133, -78.2373) -> (300.8074, -75.348)
  line L465 (300.8074, -75.348) -> (301.3128, -73.7949)
  line L466 (321.2386, -12.4725) -> (321.7492, -10.9008)
  line L467 (321.7492, -10.9008) -> (323.9585, -8.9932)
  line L468 (323.9585, -8.9932) -> (324.8501, -9.2842)
  line L469 (324.8501, -9.2842) -> (325.456, -12.1735)
  line L470 (325.456, -12.1735) -> (324.9507, -13.7266)
  line L471 (310.0202, -75.9328) -> (309.7609, -77.5626)
  line L472 (309.7609, -77.5626) -> (307.8771, -79.793)
  line L473 (307.8771, -79.793) -> (306.9511, -79.6449)
  line L474 (306.9511, -79.6449) -> (305.9007, -76.8879)
  line L475 (305.9007, -76.8879) -> (306.1573, -75.274)
  line L476 (316.2432, -11.5888) -> (316.5025, -9.9589)
  line L477 (316.5025, -9.9589) -> (318.389, -7.7285)
  line L478 (318.389, -7.7285) -> (319.3124, -7.874)
  line L479 (319.3124, -7.874) -> (320.3628, -10.6336)
  line L480 (320.3628, -10.6336) -> (320.1061, -12.2476)
  circle A90 centre (320.3628, -36.531) radius 4.019
  circle A91 centre (320.3628, -23.1193) radius 4.019
  circle A92 centre (320.3628, -64.3493) radius 4.019
  circle A93 centre (320.3628, -50.837) radius 4.019
  circle A94 centre (333.7745, -36.531) radius 4.019
  circle A95 centre (333.7745, -50.837) radius 4.019
  circle A96 centre (306.4272, -36.5337) radius 4.019
  circle A97 centre (306.4272, -23.1219) radius 4.019
  circle A98 centre (306.4272, -64.352) radius 4.019
  circle A99 centre (306.4272, -50.8423) radius 4.019
  circle A100 centre (293.0155, -36.5337) radius 4.019
  circle A101 centre (293.0155, -50.8423) radius 4.019
  line L481 (323.6542, -29.8344) -> (317.2063, -29.8344)
  line L482 (317.2063, -29.8344) -> (317.2063, -29.1333)
  arc A102 (317.2063, -29.1333) -> (314.579, -26.5086) centre (317.2037, -26.5086) cw
  spline S12 degree 3 poles (314.579, -26.5086) (314.579, -26.4636) (314.579, -26.4187) (314.579, -26.3763) knots 0 0 0 0 1 1 1 1
  line L483 (314.579, -26.3763) -> (312.1157, -26.3763)
  arc A103 (312.1157, -26.3763) -> (309.4964, -29.0063) centre (309.4911, -26.3816) cw
  line L484 (309.4964, -29.0063) -> (309.4964, -29.8397)
  line L485 (309.4964, -29.8397) -> (303.0458, -29.8397)
  arc A104 (302.9135, -29.972) -> (303.0458, -29.8397) centre (303.0458, -29.972) cw
  line L486 (302.9135, -29.972) -> (302.9135, -30.5012)
  arc A105 (303.0458, -30.6335) -> (302.9135, -30.5012) centre (303.0484, -30.4985) cw
  line L487 (303.0458, -30.6335) -> (309.4964, -30.6335)
  line L488 (309.4964, -30.6335) -> (309.4964, -31.4642)
  arc A106 (309.4964, -31.4642) -> (312.1237, -34.0916) centre (309.4964, -34.0916) cw
  line L489 (312.1237, -34.0916) -> (314.579, -34.0916)
  arc A107 (314.579, -34.0916) -> (317.2063, -31.4643) centre (317.2063, -34.0916) cw
  line L490 (317.2063, -31.4643) -> (317.2063, -30.6335)
  line L491 (317.2063, -30.6335) -> (323.6542, -30.6335)
  arc A108 (323.7865, -30.5012) -> (323.6542, -30.6335) centre (323.6542, -30.5012) cw
  line L492 (323.7865, -30.5012) -> (323.7865, -29.972)
  arc A109 (323.6542, -29.8344) -> (323.7865, -29.972) centre (323.6543, -29.9667) cw
  line L493 (323.6542, -57.5178) -> (317.2063, -57.5178)
  line L494 (317.2063, -57.5178) -> (317.2063, -56.8193)
  arc A110 (317.2063, -56.8193) -> (314.579, -54.192) centre (317.2063, -54.192) cw
  spline S13 degree 3 poles (314.579, -54.192) (314.579, -54.147) (314.579, -54.1046) (314.579, -54.0597) knots 0 0 0 0 1 1 1 1
  line L495 (314.579, -54.0597) -> (312.1157, -54.0597)
  arc A111 (312.1157, -54.0597) -> (309.4884, -56.687) centre (309.4884, -54.0597) cw
  line L496 (309.4884, -56.687) -> (309.4884, -57.5178)
  line L497 (309.4884, -57.5178) -> (303.0458, -57.5178)
  arc A112 (302.9135, -57.6501) -> (303.0458, -57.5178) centre (303.0484, -57.6527) cw
  line L498 (302.9135, -57.6501) -> (302.9135, -58.1792)
  arc A113 (303.0458, -58.3115) -> (302.9135, -58.1792) centre (303.0484, -58.1766) cw
  line L499 (303.0458, -58.3115) -> (309.4964, -58.3115)
  line L500 (309.4964, -58.3115) -> (309.4964, -59.1423)
  arc A114 (309.4964, -59.1423) -> (312.1237, -61.7696) centre (309.4964, -61.7696) cw
  line L501 (312.1237, -61.7696) -> (314.579, -61.7696)
  arc A115 (314.579, -61.7696) -> (317.2063, -59.1423) centre (317.2063, -61.7696) cw
  line L502 (317.2063, -59.1423) -> (317.2063, -58.3115)
  line L503 (317.2063, -58.3115) -> (323.6542, -58.3115)
  arc A116 (323.7865, -58.1792) -> (323.6542, -58.3115) centre (323.6542, -58.1792) cw
  line L504 (323.7865, -58.1792) -> (323.7865, -57.6501)
  arc A117 (323.6542, -57.5178) -> (323.7865, -57.6501) centre (323.6542, -57.6501) cw
  line L505 (299.1141, -33.7688) -> (299.1141, -40.2193)
  line L506 (299.1141, -40.2193) -> (298.413, -40.2193)
  arc A118 (298.413, -40.2193) -> (295.7856, -42.8466) centre (295.7883, -40.222) cw
  line L507 (295.7856, -42.8466) -> (295.6534, -42.8466)
  line L508 (295.6534, -42.8466) -> (295.6534, -45.3073)
  arc A119 (295.6534, -45.3073) -> (298.2807, -47.9346) centre (295.656, -47.9319) cw
  line L509 (298.2807, -47.9346) -> (299.1141, -47.9346)
  line L510 (299.1141, -47.9346) -> (299.1141, -54.3851)
  arc A120 (299.2464, -54.5174) -> (299.1141, -54.3851) centre (299.2464, -54.3851) cw
  line L511 (299.2464, -54.5174) -> (299.7756, -54.5174)
  arc A121 (299.9079, -54.3851) -> (299.7756, -54.5174) centre (299.7756, -54.3851) cw
  line L512 (299.9079, -54.3851) -> (299.9079, -47.9266)
  line L513 (299.9079, -47.9266) -> (300.7386, -47.9266)
  arc A122 (300.7386, -47.9266) -> (303.366, -45.2993) centre (303.366, -47.9266) cw
  line L514 (303.366, -45.2993) -> (303.366, -42.844)
  arc A123 (303.366, -42.844) -> (300.7386, -40.2167) centre (303.366, -40.2167) cw
  line L515 (300.7386, -40.2167) -> (299.9052, -40.2167)
  line L516 (299.9052, -40.2167) -> (299.9052, -33.7688)
  arc A124 (299.7729, -33.6365) -> (299.9052, -33.7688) centre (299.7729, -33.7688) cw
  line L517 (299.7729, -33.6365) -> (299.2438, -33.6365)
  arc A125 (299.1141, -33.7688) -> (299.2438, -33.6365) centre (299.2464, -33.7687) cw
  line L518 (326.7975, -33.7688) -> (326.7975, -40.2193)
  line L519 (326.7975, -40.2193) -> (326.099, -40.2193)
  arc A126 (326.099, -40.2193) -> (323.4716, -42.8466) centre (323.4716, -40.2193) cw
  line L520 (323.4716, -42.8466) -> (323.3394, -42.8466)
  line L521 (323.3394, -42.8466) -> (323.3394, -45.3073)
  arc A127 (323.3394, -45.3073) -> (325.9667, -47.9346) centre (323.3394, -47.9346) cw
  line L522 (325.9667, -47.9346) -> (326.7975, -47.9346)
  line L523 (326.7975, -47.9346) -> (326.7975, -54.3851)
  arc A128 (326.9298, -54.5174) -> (326.7975, -54.3851) centre (326.9324, -54.3825) cw
  line L524 (326.9298, -54.5174) -> (327.4589, -54.5174)
  arc A129 (327.5912, -54.3851) -> (327.4589, -54.5174) centre (327.4563, -54.3825) cw
  line L525 (327.5912, -54.3851) -> (327.5912, -47.9266)
  line L526 (327.5912, -47.9266) -> (328.422, -47.9266)
  arc A130 (328.422, -47.9266) -> (331.0493, -45.2993) centre (331.0493, -47.9266) cw
  line L527 (331.0493, -45.2993) -> (331.0493, -42.844)
  arc A131 (331.0493, -42.844) -> (328.422, -40.2167) centre (331.0493, -40.2167) cw
  line L528 (328.422, -40.2167) -> (327.5912, -40.2167)
  line L529 (327.5912, -40.2167) -> (327.5912, -33.7688)
  arc A132 (327.4589, -33.6365) -> (327.5912, -33.7688) centre (327.4563, -33.7714) cw
  line L530 (327.4589, -33.6365) -> (326.9298, -33.6365)
  arc A133 (326.7975, -33.7688) -> (326.9298, -33.6365) centre (326.9324, -33.7714) cw
  line L531 (314.3885, -39.9071) -> (313.9202, -39.9071)
  line L532 (313.9202, -39.9071) -> (313.9202, -35.777)
  arc A134 (313.7879, -35.6447) -> (313.9202, -35.777) centre (313.7879, -35.777) cw
  line L533 (313.7879, -35.6447) -> (312.6925, -35.6447)
  arc A135 (312.5602, -35.777) -> (312.6925, -35.6447) centre (312.6951, -35.7796) cw
  line L534 (312.5602, -35.777) -> (312.5602, -39.9071)
  line L535 (312.5602, -39.9071) -> (312.0655, -39.9071)
  arc A136 (312.0655, -39.9071) -> (309.4381, -42.5344) centre (309.4381, -39.9071) cw
  spline S14 degree 3 poles (309.4381, -42.5344) (309.3932, -42.5344) (309.3508, -42.5344) (309.3059, -42.5344) knots 0 0 0 0 1 1 1 1
  line L536 (309.3059, -42.5344) -> (309.3059, -44.995)
  arc A137 (309.3059, -44.995) -> (311.9332, -47.6224) centre (309.3059, -47.6224) cw
  line L537 (311.9332, -47.6224) -> (312.5602, -47.6224)
  line L538 (312.5602, -47.6224) -> (312.5602, -51.7049)
  arc A138 (312.6925, -51.8372) -> (312.5602, -51.7049) centre (312.6951, -51.7023) cw
  line L539 (312.6925, -51.8372) -> (313.7879, -51.8372)
  arc A139 (313.9202, -51.7049) -> (313.7879, -51.8372) centre (313.7879, -51.7049) cw
  line L540 (313.9202, -51.7049) -> (313.9202, -47.6144)
  line L541 (313.9202, -47.6144) -> (314.3885, -47.6144)
  arc A140 (314.3885, -47.6144) -> (317.0158, -44.9871) centre (317.0158, -47.6144) cw
  line L542 (317.0158, -44.9871) -> (317.0158, -42.5344)
  arc A141 (317.0158, -42.5344) -> (314.3885, -39.9071) centre (317.0158, -39.9071) cw
  arc A142 (320.3522, -17.8938) -> (324.0564, -26.8129) centre (320.3664, -23.1166) cw
  spline S15 degree 3 poles (320.3522, -17.8938) (317.4656, -17.8938) (315.1505, -20.275) (315.1637, -23.45) knots 0 0 0 0 1 1 1 1
  spline S16 degree 3 poles (315.1373, -64.9208) (315.1373, -67.8048) (317.4762, -69.5748) (320.3628, -69.5748) knots 0 0 0 0 1 1 1 1
  arc A143 (324.0431, -60.6399) -> (320.3628, -69.5748) centre (320.3627, -64.3493) cw
  arc A144 (330.0704, -32.8348) -> (333.7745, -41.7565) centre (333.7641, -36.531) cw
  arc A145 (333.7745, -45.6115) -> (330.0915, -54.5465) centre (333.772, -50.837) cw
  arc A146 (301.0032, -64.352) -> (302.4055, -60.6928) centre (306.6491, -64.4173) cw
  arc A147 (306.2314, -69.5775) -> (301.0032, -64.352) centre (306.2314, -64.3493) cw
  spline S17 degree 3 poles (306.2314, -69.5775) (309.1048, -69.5775) (311.3961, -67.4793) (311.4887, -64.815) knots 0 0 0 0 1 1 1 1
  arc A148 (287.7899, -36.5443) -> (296.709, -32.8401) centre (293.0128, -36.5301) cw
  spline S18 degree 3 poles (287.7899, -36.5443) (287.7899, -39.4309) (289.9675, -41.7698) (292.8514, -41.7698) knots 0 0 0 0 1 1 1 1
  spline S19 degree 3 poles (292.7456, -45.5904) (289.859, -45.5904) (287.7899, -47.9557) (287.7899, -50.8423) knots 0 0 0 0 1 1 1 1
  arc A149 (296.6191, -54.6206) -> (287.7899, -50.8423) centre (293.0102, -50.8488) cw
  arc A150 (302.641, -26.9081) -> (311.494, -23.1219) centre (306.2499, -23.1035) cw
  line L543 (302.641, -26.9081) -> (296.709, -32.8374)
  line L544 (324.0564, -26.8129) -> (330.0783, -32.8348)
  line L545 (324.0431, -60.6399) -> (330.0942, -54.5465)
  line L546 (302.4055, -60.6928) -> (296.6191, -54.6206)
  spline S20 degree 3 poles (311.494, -23.1219) (311.494, -24.2305) (312.2454, -25.1301) (313.1767, -25.1381) knots 0 0 0 0 1 1 1 1
  line L547 (313.1741, -25.1381) -> (313.1899, -25.1381)
  spline S21 degree 3 poles (313.1741, -25.1381) (314.2059, -25.1381) (315.05, -24.4713) (315.1584, -23.6273) knots 0 0 0 0 1 1 1 1
  line L548 (313.1741, -25.1381) -> (313.1555, -25.1381)
  arc A151 (315.1743, -23.4421) -> (315.1611, -23.6273) centre (313.7218, -23.4314) cw
  spline S22 degree 3 poles (315.1743, -65.3574) (315.1743, -64.2488) (314.4229, -63.3492) (313.4916, -63.3413) knots 0 0 0 0 1 1 1 1
  arc A152 (311.494, -64.9896) -> (311.6501, -64.3758) centre (312.7931, -64.9932) cw
  arc A153 (311.6395, -64.3811) -> (313.4916, -63.3412) centre (313.4212, -65.3853) cw
  line L549 (313.4916, -63.3413) -> (313.5101, -63.3412)
  arc A154 (294.2325, -43.8256) -> (292.4149, -45.6168) centre (292.4519, -43.8366) cw
  line L550 (294.2325, -43.8441) -> (294.2325, -43.8229)
  spline S23 degree 3 poles (292.6953, -41.7486) (293.6266, -41.7486) (294.2246, -42.7196) (294.2325, -43.8256) knots 0 0 0 0 1 1 1 1
  spline S24 degree 3 poles (333.7745, -41.7565) (332.8643, -41.7565) (332.2532, -42.5794) (332.2452, -43.5107) knots 0 0 0 0 1 1 1 1
  spline S25 degree 3 poles (333.7745, -45.6115) (332.6024, -45.6115) (332.2532, -44.6167) (332.2452, -43.5107) knots 0 0 0 0 1 1 1 1
  arc A155 (336.1425, -23.4659) -> (336.0817, -64.0794) centre (313.1977, -43.7383) cw
  line L551 (336.0817, -64.0794) -> (328.3267, -56.3245)
  arc A156 (292.8488, -20.8465) -> (333.4438, -20.7671) centre (313.1911, -43.7329) cw
  line L552 (292.8488, -20.8465) -> (300.7863, -28.784)
  line L553 (333.4438, -20.7671) -> (325.7285, -28.485)
  line L554 (336.1452, -23.4659) -> (328.4273, -31.1811)
  line L555 (298.0769, -31.4695) -> (290.1553, -23.5532)
  arc A157 (290.2162, -63.9895) -> (290.1553, -23.5532) centre (313.1819, -43.7367) cw
  line L556 (290.2162, -63.9895) -> (298.0637, -56.1419)
  line L557 (300.7042, -58.9042) -> (292.9202, -66.6882)
  arc A158 (333.375, -66.7676) -> (292.9202, -66.6882) centre (313.1927, -43.7435) cw
  line L558 (333.375, -66.7676) -> (325.6386, -59.0338)
  line L559 (296.709, -32.8374) -> (298.0769, -31.4695)
  line L560 (298.0769, -31.4695) -> (302.641, -26.9081)
  point P0 (68.8102, -36.5204)
  point P1 (47.7917, -29.3132)
  point P2 (47.7917, -15.9015)
  point P3 (47.7917, -57.1315)
  point P4 (47.7917, -43.6219)
  point P5 (61.2034, -29.3132)
  point P6 (61.2034, -43.6219)
  point P7 (33.8561, -29.3158)
  point P8 (33.8561, -15.9041)
  point P9 (33.8561, -57.1341)
  point P10 (33.8561, -43.6245)
  point P11 (20.4444, -29.3158)
  point P12 (20.4444, -43.6245)
  point P13 (33.6656, -15.9041)
  point P14 (345.3977, -43.7383)
  point P15 (324.3818, -36.531)
  point P16 (324.3818, -23.1193)
  point P17 (324.3818, -64.3493)
  point P18 (324.3818, -50.837)
  point P19 (337.7935, -36.531)
  point P20 (337.7935, -50.837)
  point P21 (310.4462, -36.5337)
  point P22 (310.4462, -23.1219)
  point P23 (310.4462, -64.352)
  point P24 (310.4462, -50.8423)
  point P25 (297.0345, -36.5337)
  point P26 (297.0345, -50.8423)